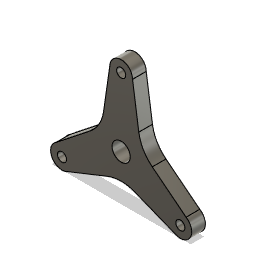
Stern (Autodesk Fusion 360 design; units mm, degrees)
Autodesk Fusion 360 part; units mm, degrees
sketch "Skizze1" plane through (0, 0, 0) normal (0, 0, 1) x (1, 0, 0)
  circle A0 centre (0, 0) radius 25
  circle A1 centre (0, 75) radius 12.5
  line L0 (0, 0) -> (21.6506, 12.5) construction
  line L1 (0, 0) -> (25, 0) construction
  line L2 (21.6506, 12.5) -> (12.5, 75)
  line L3 (0, 0) -> (-21.6506, 12.5) construction
  line L4 (-21.6506, 12.5) -> (-12.5, 75)
  line L5 (0, 75) -> (0, 0) construction
  line L6 (0, 75) -> (-12.5, 75) construction
  line L7 (0, 75) -> (12.5, 75) construction
  line L8 (-21.6506, 12.5) -> (-71.2019, -26.6747)
  circle A2 centre (-64.9519, -37.5) radius 12.5
  line L9 (0, -25) -> (-58.7019, -48.3253)
  line L10 (0, -25) -> (58.7019, -48.3253)
  circle A3 centre (64.9519, -37.5) radius 12.5
  line L11 (21.6506, 12.5) -> (71.2019, -26.6747)
  dimension "d1" = 50
  dimension "d3" = 25
  dimension "d4" = 30
  dimension "d5" = 30
  dimension "d6" = 75
  dimension "d10" = 360
  constraint horizontal L1
  constraint coincident A0.centre L0.start
  constraint coincident A0 L0.end
  constraint coincident A1 L2.end
  constraint coincident A0 L3.end
  constraint coincident A1 L4.end
  constraint coincident A1.centre L5.start
  constraint perpendicular L1 L5
  constraint perpendicular L5 L6
  constraint perpendicular L5 L7
  constraint coincident L2.end L7.end
  constraint coincident L4.end L6.end
  measures "d1" diameter of A0
  measures "d3" diameter of A1
  measures "d4" angle of L0 L1
  measures "d5" angle of L1 L3
  measures "d6" distance of A1.centre A0.centre
extrude "Extrusion1" add sketch "Skizze1" along normal blind 15
fillet "Abrundung1" radius 40 3 edges at (-21.6506, 12.5, 7.5) (0, -25, 7.5) (21.6506, 12.5, 7.5)
sketch "Skizze2" plane through (0, 0, 0) normal (0, 0, -1) x (-1, 0, 0)
  arc A0 (12.5, 75) -> (-12.5, 75) centre (0, 75) ccw
  line L0 (-12.5, 75) -> (-19.3481, 28.2264)
  arc A1 (-34.1189, 2.6428) -> (-19.3481, 28.2264) centre (-58.9262, 34.021) ccw
  line L1 (-34.1189, 2.6428) -> (-71.2019, -26.6747)
  arc A2 (-71.2019, -26.6747) -> (-58.7019, -48.3253) centre (-64.9519, -37.5) ccw
  line L2 (-58.7019, -48.3253) -> (-14.7707, -30.8692)
  arc A3 (14.7707, -30.8692) -> (-14.7707, -30.8692) centre (0, -68.0421) ccw
  line L3 (14.7707, -30.8692) -> (58.7019, -48.3253)
  arc A4 (58.7019, -48.3253) -> (71.2019, -26.6747) centre (64.9519, -37.5) ccw
  line L4 (71.2019, -26.6747) -> (34.1189, 2.6428)
  arc A5 (19.3481, 28.2264) -> (34.1189, 2.6428) centre (58.9262, 34.021) ccw
  line L5 (19.3481, 28.2264) -> (12.5, 75)
  point P0 (0, 75)
  point P1 (-64.9519, -37.5)
  point P2 (64.9519, -37.5)
  constraint coincident P0 A0.centre
  constraint coincident P1 A2.centre
  constraint coincident P2 A4.centre
hole "Bohrung1" at (0, 75, 0) at (-64.9519, -37.5, 0) at (64.9519, -37.5, 0) direction (0, 0, 1) diameter 10 end through all
sketch "Skizze4" plane through (0, 0, 0) normal (0, 0, -1) x (-1, 0, 0)
  circle A0 centre (64.9519, -37.5) radius 5
  circle A1 centre (0, 75) radius 5
  circle A2 centre (-64.9519, -37.5) radius 5
  arc A3 (12.5, 75) -> (-12.5, 75) centre (0, 75) ccw
  line L0 (-12.5, 75) -> (-19.3481, 28.2264)
  arc A4 (-34.1189, 2.6428) -> (-19.3481, 28.2264) centre (-58.9262, 34.021) ccw
  line L1 (-34.1189, 2.6428) -> (-71.2019, -26.6747)
  arc A5 (-71.2019, -26.6747) -> (-58.7019, -48.3253) centre (-64.9519, -37.5) ccw
  line L2 (-58.7019, -48.3253) -> (-14.7707, -30.8692)
  arc A6 (14.7707, -30.8692) -> (-14.7707, -30.8692) centre (0, -68.0421) ccw
  line L3 (14.7707, -30.8692) -> (58.7019, -48.3253)
  arc A7 (58.7019, -48.3253) -> (71.2019, -26.6747) centre (64.9519, -37.5) ccw
  line L4 (71.2019, -26.6747) -> (34.1189, 2.6428)
  arc A8 (19.3481, 28.2264) -> (34.1189, 2.6428) centre (58.9262, 34.021) ccw
  line L5 (19.3481, 28.2264) -> (12.5, 75)
hole "Bohrung2" at (0, 0, 0) direction (0, 0, 1) diameter 20 end through all
